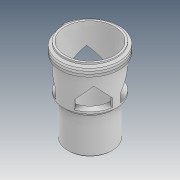
# Autodesk Inventor part: PMBase
Saved by Autodesk Inventor 2020 (Build 240168000, 168)
## iProperties
Created: 2020-05-07
Part Number: PMBase
Material: Generic
Document SubType Name: Modeling
Designer: Theo Cominotto
Density: 1 g/cm^3
Appearance: Default
ThreadHeight: 1,400 mm
ThreadPitch: 1,250 mm
Author: Theo Cominotto
Autodesk Inventor part; units mm, degrees
ref_plane "YZ Plane" through (0, 0, 0) normal (1, 0, 0) x (0, 1, 0)
ref_plane "XZ Plane" through (0, 0, 0) normal (0, 1, 0) x (-1, 0, 0)
sketch "Sketch1" plane through (0, 0, 0) normal (0, 0, 1) x (1, 0, 0)
  line L0 (0, 0) -> (0, 20) construction
  line L1 (0, 20) -> (11.2, 20) construction
  line L2 (11.2, 20) -> (11, 0)
  line L3 (11, 0) -> (0, 0) construction
  line L4 (11, 0) -> (9.8, 0)
  line L5 (11, 0) -> (12.2, 0) construction
  line L6 (9.8, 0) -> (9.8, 20)
  line L7 (9.8, 20) -> (11.2, 20)
  dimension "d0" = 20
  dimension "d1" = 11.2
  dimension "d2" = 11
  dimension "d4" = 180
  dimension "d9" = 9.8
  constraints: 16 end point, 3 perpendicular, 2 collinear, 1 horizontal, 1 parallel, 1 point on line, 1 vertical
  measures "d0" distance of L0.start L0.end
  measures "d1" distance of L0.end L1.end
  measures "d2" distance of L2.end L0.start
  measures "d4" angle of L5 L4
  measures "d9" distance between parallel lines of L0 L6
revolve "Revolution1" add sketch "Sketch1" angle 360 about axis through (0, 0, 0) along (0, 1, 0)
chamfer "Chamfer1" distance 0.6 angle 45 1 edges at (-11, 0, 0)
sketch "Sketch2" plane through (0, 20, 0) normal (0, 1, 0) x (1, 0, 0)
  circle A0 centre (0, 0) radius 13.2
  circle A1 centre (0, 0) radius 9.8 projected
  dimension "d10" = 26.4
  constraints: 1 centre point, 1 coincident
  measures "d10" diameter of A0
extrude "Extrusion1" add sketch "Sketch2" along normal blind 1
chamfer "Chamfer2" distance 2 angle 45 1 edges at (-11.2, 20, 0)
sketch "Sketch3" plane through (0, 21, 0) normal (0, 1, 0) x (1, 0, 0)
  circle A0 centre (0, 0) radius 13.2 projected
  circle A1 centre (0, 0) radius 12.25
  line L0 (0, 0) -> (4.5, 12.4093)
  line L1 (0, 0) -> (-4.5, 12.4093)
  line L2 (-18.48, 0) -> (18.48, 0) construction
  line L3 (0, 18.48) -> (0, -18.48) construction
  line L4 (0, 0) -> (4.5, -12.4093)
  line L5 (0, 0) -> (-4.5, -12.4093)
  line L6 (0, 0) -> (13.0476, 2)
  line L7 (0, 0) -> (13.0476, -2)
  line L8 (0, 0) -> (-13.0476, 2)
  line L9 (0, 0) -> (-13.0476, -2)
  point P0 (-4.1761, -11.5162)
  point P1 (4.1761, -11.5162)
  point P2 (12.1086, -1.8561)
  point P3 (12.1086, 1.8561)
  point P4 (-4.1761, 11.5162)
  point P5 (4.1761, 11.5162)
  point P6 (-12.1086, 1.8561)
  point P7 (-12.1086, -1.8561)
  dimension "d16" = 24.5
  dimension "d17" = 9
  dimension "d18" = 4
  constraints: 16 end point, 5 symmetric about line, 3 point on circle, 1 centre point, 1 coincident, 1 other
  measures "d16" diameter of A1
  measures "d17" distance of L0.end L1.end
  measures "d18" distance of L7.end L6.end
extrude "Extrusion2" add sketch "Sketch3" along normal blind 11 contours A0 L7 A1 L6 | L0 A1 L1 A0 | A0 L5 A1 L4 | L8 A1 L9 A0
sketch "Sketch4" plane through (0, 32, 0) normal (0, 1, 0) x (1, 0, 0)
  circle A0 centre (0, 0) radius 13.2
  circle A1 centre (0, 0) radius 12.25
  arc A2 (-4.5, 12.4093) -> (-13.0476, 2) centre (0, 0) ccw projected
  arc A3 (4.1761, 11.5162) -> (-4.1761, 11.5162) centre (0, 0) ccw projected
  constraints: 2 centre point, 2 coincident, 2 concentric
extrude "Extrusion3" add sketch "Sketch4" along normal blind 10
chamfer "Chamfer3" distance 6.73 angle 45 8 edges at (-4.3381, 32, 11.9627) (-12.5781, 32, 1.928) (4.3381, 32, 11.9627) (12.5781, 32, 1.928) (12.5781, 32, -1.928) (4.3381, 32, -11.9627) (-4.3381, 32, -11.9627) (-12.5781, 32, -1.928)
sketch "Sketch5" plane through (0, 0, 0) normal (0, 0, 1) x (1, 0, 0)
  line L0 (-13.2, 20) -> (-13.2, 42) projected
  line L1 (-13.2, 42) -> (-14.6, 41.375)
  line L2 (-14.6, 41.375) -> (-13.2, 40.75)
  line L3 (-14.6, 41.375) -> (-13.2, 41.375) construction
  line L4 (13.2, 42) -> (-13.2, 42) projected
  point P0 (0, 0)
  dimension "d27" = 1.25
  dimension "d55" = 1.4
  constraints: 6 end point, 4 point on line, 1 perpendicular, 1 other
  measures "d27" distance of L1.start L2.end
  measures "d55" distance of L1.end L3.end
ref_plane "Work Plane1" through (0, 41.375, 0) normal (0, 1, 0) x (1, 0, 0)
coil "Coil3" sketch "Sketch5" operation add axis through (0, -10, 0) along (0, -1, 0) pitch 1.25 turns 4 hand right
chamfer "Chamfer5" distance 0.559 angle 45 4 edges at (-13.9, 41.6875, 0) (-13.9, 41.0625, 0) (-13.9, 36.6875, 0) (-13.9, 36.0625, 0)
equation "\"d27\" = ThreadPitch"
equation "\"d55\" = ThreadHeight"
equation "\"d56\" = ThreadPitch"
equation "\"ThreadHeight\" = 1.4"
equation "\"ThreadPitch\" = 1.25"
equation "\"d36\" = -0.5 * ThreadPitch"
body "Solid1"
